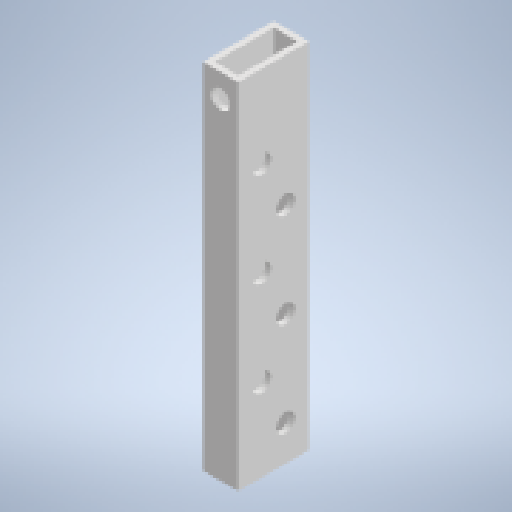
# Autodesk Inventor part: hinge base
Saved by Autodesk Inventor 2025.2 (Build 292293000, 293)
## iProperties
Created: 2025-01-08
Part Number: hinge base
Material: Generic
Document SubType Name: Modeling
Designer: 5013908
Density: 1 g/cm^3
Appearance: Default
Author: 5013908
Autodesk Inventor part; units mm, degrees
ref_plane "YZ Plane" through (0, 0, 0) normal (1, 0, 0) x (0, 1, 0)
ref_plane "XZ Plane" through (0, 0, 0) normal (0, 1, 0) x (-1, 0, 0)
ref_plane "XY Plane" through (0, 0, 0) normal (0, 0, 1) x (1, 0, 0)
sketch "Sketch1" plane through (0, 0, 0) normal (0, 1, 0) x (-1, 0, 0)
  line L0 (0, 0) -> (19.05, 0)
  line L1 (19.05, 0) -> (19.05, -38.1)
  line L2 (19.05, -38.1) -> (0, -38.1)
  line L3 (0, -38.1) -> (0, 0)
  line L4 (15.875, -34.925) -> (15.875, -3.175)
  line L5 (15.875, -3.175) -> (3.175, -3.175)
  line L6 (3.175, -3.175) -> (3.175, -34.925)
  line L7 (3.175, -34.925) -> (15.875, -34.925)
  dimension "d0" = 19.05
  dimension "d1" = 38.1
  dimension "d2" = 3.175
  constraints: 16 end point, 4 parallel, 2 perpendicular, 1 horizontal, 3 other
  measures "d0" distance of L1.end L2.end
  measures "d1" distance of L0.end L1.end
  measures "d2" distance between parallel lines of L1 L4
extrude "Extrusion1" add sketch "Sketch1" along normal blind 190.5
sketch "Sketch2" plane through (-19.05, 0, 0) normal (0, 0, 1) x (1, 0, 0)
  circle A0 centre (9.525, 177.8) radius 5
  line L0 (15.875, 0) -> (15.875, 190.5) projected
  line L1 (0, 0) -> (19.05, 0) projected
  line L2 (19.05, 0) -> (19.05, 190.5) projected
  line L3 (0, 190.5) -> (19.05, 190.5) projected
  line L4 (0, 0) -> (0, 190.5) projected
  point P0 (9.525, 190.5)
  dimension "d5" = 10
  dimension "d6" = 9.525
  dimension "d7" = 12.7
  constraints: 1 centre point, 1 midpoint
  measures "d5" diameter of A0
  measures "d6" distance from line of L4 A0.centre
  measures "d7" distance of point (9.525, 190.5) A0.centre
extrude "Extrusion2" cut sketch "Sketch2" against normal blind 204.7875 contours A0
sketch "Sketch3" plane through (0, 0, 0) normal (1, 0, 0) x (0, 0, -1)
  line L0 (25.3873, 190.5) -> (25.3873, 0)
  line L1 (38.1, 190.5) -> (38.1, 0)
  line L2 (38.1, 0) -> (0, 0) projected
  line L3 (38.1, 190.5) -> (25.3873, 190.5)
  line L4 (38.1, 0) -> (38.1, 190.5) projected
  line L5 (25.3873, 190.5) -> (38.1, 190.5)
  line L6 (38.1, 190.5) -> (0, 190.5)
  line L7 (0, 190.5) -> (38.1, 190.5) projected
  line L8 (12.6873, 190.5) -> (12.6873, 0)
  circle A0 centre (25.3873, 19.05) radius 5
  circle A1 centre (12.6873, 44.45) radius 5
  circle A2 centre (25.3873, 69.85) radius 5
  circle A3 centre (25.3873, 120.65) radius 5
  circle A4 centre (12.6873, 95.25) radius 5
  circle A5 centre (12.6873, 146.05) radius 5
  dimension "d10" = 12.7
  dimension "d11" = 10
  dimension "d12" = 10
  dimension "d15" = 50.8
  dimension "d20" = 19.05
  dimension "d21" = 25.4
  dimension "d24" = 50.8
  constraints: 12 end point, 6 centre point, 5 point on line, 3 vertical, 2 collinear, 2 perpendicular, 8 other
  measures "d10" distance between parallel lines of L0 L8
  measures "d11" diameter of A0
  measures "d12" diameter of A1
  measures "d15" distance of A0.centre A2.centre
  measures "d20" distance from line of L2 A0.centre
  measures "d21" vertical distance of A0.centre A1.centre
  measures "d24" distance of A1.centre A4.centre
extrude "Extrusion3" cut sketch "Sketch3" against normal blind 204.7875 contours A3 L0 | L0 A3 | A5 L8 | L8 A5 | A2 L0 | L0 A2 | A0 L0 | L0 A0 | A4 L8 | L8 A4 | A1 L8 | L8 A1
body "Solid1"
